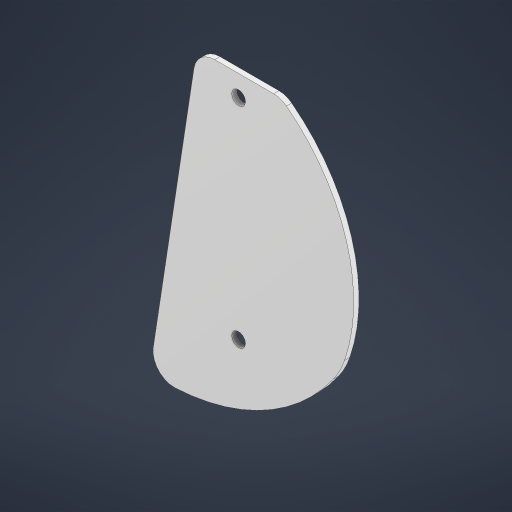
# Autodesk Inventor part: sled
Saved by Autodesk Inventor 2024 (Build 280153000, 153)
## iProperties
Created: 2023-10-27
Part Number: sled
Material: Acetal Resin, White
Document SubType Name: Modeling
Designer: Averey Ku
Density: 1.425 g/cm^3
Appearance: Smooth - White
Author: Averey Ku
Autodesk Inventor part; units mm, degrees
ref_plane "YZ Plane" through (0, 0, 0) normal (1, 0, 0) x (0, 1, 0)
ref_plane "XZ Plane" through (0, 0, 0) normal (0, 1, 0) x (-1, 0, 0)
ref_plane "XY Plane" through (0, 0, 0) normal (0, 0, 1) x (1, 0, 0)
sketch "Sketch1" plane through (0, 0, 0) normal (0, 0, 1) x (1, 0, 0)
  circle A0 centre (-26.9881, -17.2743) radius 2.0955
  circle A1 centre (-26.9881, 46.2257) radius 2.0955
  arc A2 (-46.2652, -39.5915) -> (1.8146, -13.1917) centre (-49.3718, 23.0479) ccw
  arc A3 (5.1303, -6.697) -> (-12.4868, 51.2687) centre (-44.0163, 10.0263) ccw
  line L0 (-52.8546, -32.2756) -> (-40.5223, 47.1977)
  line L1 (-34.2474, 52.574) -> (-16.3434, 52.574)
  arc A4 (1.8146, -13.1917) -> (5.1303, -6.697) centre (-18.9158, 1.4852) ccw
  arc A5 (-52.8546, -32.2756) -> (-46.2652, -39.5915) centre (-46.5797, -33.2493) ccw
  arc A6 (-34.2474, 52.574) -> (-40.5223, 47.1977) centre (-34.2474, 46.224) ccw
  arc A7 (-12.4868, 51.2687) -> (-16.3434, 52.574) centre (-16.3434, 46.224) ccw
  point P0 (-53.9756, -39.4993)
  point P1 (-14.2718, 52.574)
  dimension "d5" = 4.191
  dimension "d6" = 4.191
  dimension "d7" = 25.4
  dimension "d8" = 6.35
  dimension "d9" = 6.35
  constraints: 14 point on circle, 8 centre point, 8 tangent, 4 end point, 2 point on line, 1 equal radius, 1 horizontal
  measures "d5" diameter of A0
  measures "d6" diameter of A1
  measures "d7" radius of A4
  measures "d8" radius of A5
  measures "d9" radius of A6
extrude "Extrusion1" add sketch "Sketch1" along normal blind 1.5875
body "Solid1"
